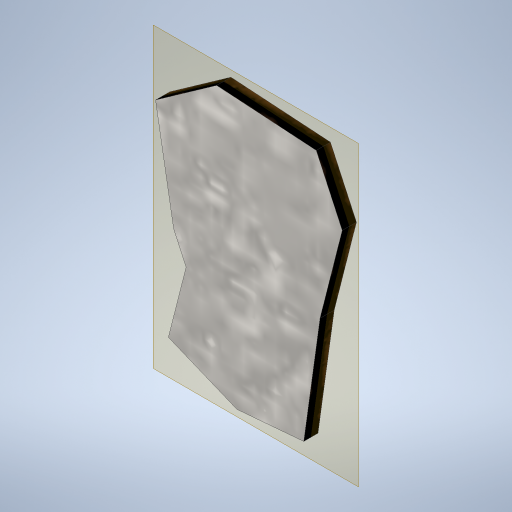
# Autodesk Inventor part: emu
Saved by Autodesk Inventor 2023 (Build 270158000, 158)
## iProperties
Created: 2024-07-02
Part Number: emu
Material: Generic
Document SubType Name: Modeling
Designer: Student-27
Density: 1 g/cm^3
Appearance: Default
Author: Student-27
Autodesk Inventor part; units mm, degrees
ref_plane "YZ Plane" through (0, 0, 0) normal (1, 0, 0) x (0, 1, 0)
ref_plane "XZ Plane" through (0, 0, 0) normal (0, 1, 0) x (-1, 0, 0)
sketch "Sketch1" plane through (0, 0, 0) normal (0, 0, 1) x (1, 0, 0)
  line L0 (721.6141, 114.4876) -> (1521.7141, 114.4876) construction
  line L1 (1521.7141, 114.4876) -> (1521.7141, -952.3124) construction
  line L2 (1521.7141, -952.3124) -> (721.6141, -952.3124) construction
  line L3 (721.6141, -952.3124) -> (721.6141, 114.4876) construction
  line L4 (-7.056, 29.0093) -> (14.3013, 27.6134)
  line L5 (14.3013, 27.6134) -> (19.8775, 15.5316)
  line L6 (19.8775, 15.5316) -> (15.1145, -3.1721)
  line L7 (15.1145, -3.1721) -> (11.6293, -27.8005)
  line L8 (11.6293, -27.8005) -> (-2.7232, -29.0093)
  line L9 (-2.7232, -29.0093) -> (-17.4171, -22.9801)
  line L10 (-17.4171, -22.9801) -> (-13.6138, -8.0453)
  line L11 (-13.6138, -8.0453) -> (-16.2905, -2.2458)
  line L12 (-16.2905, -2.2458) -> (-20.1715, 19.7348)
  line L13 (-20.1715, 19.7348) -> (-7.056, 29.0093)
  line L14 (-20.1715, 29.0093) -> (20.1637, 29.0093)
  line L15 (20.1637, 29.0093) -> (20.1637, -29.0093)
  line L16 (20.1637, -29.0093) -> (-20.1715, -29.0093)
  line L17 (-20.1715, -29.0093) -> (-20.1715, 29.0093)
  point P0 (0, 0)
  point P1 (0, 0)
  dimension "d7" = 40.3352
  dimension "d10" = 58.0187
  constraints: 28 end point, 4 parallel, 1 horizontal, 1 perpendicular, 2 other
  measures "d7" distance of L14.start L14.end
  measures "d10" distance of L16.end L14.start
extrude "Extrusion1" add sketch "Sketch1" along normal mid plane 3.048 contours L4 L5 L6 L7 L8 L9 L10 L11 L12 L13
body "Solid1"
